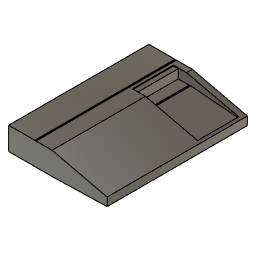
Basic shape (no keyboardd) hahahahahahah v1 (Autodesk Fusion 360 design; units mm, degrees)
Autodesk Fusion 360 part; units mm, degrees
sketch "Sketch1" plane through (0, 0, 0) normal (0, 1, 0) x (1, 0, 0)
  line L0 (0, 0) -> (0, -60.3)
  line L1 (0, 0) -> (115, 0)
  line L2 (0, -60.3) -> (115, -60.3)
  line L3 (261, -25.8907) -> (261, -3.8907)
  line L4 (115, 0) -> (261, -3.8907)
  line L5 (261, -25.8907) -> (115, -60.3)
  dimension "d1" = 60.3
  dimension "d2" = 115
  dimension "d3" = 115
  dimension "d4" = 150
  dimension "d5" = 22
  dimension "d6" = 146
  constraint coincident L0.start L1.start
  constraint vertical L0
  constraint perpendicular L0 L1
  constraint perpendicular L0 L2
  constraint vertical L3
  measures "d1" distance of L0.start L0.end
  measures "d2" distance of L0.start L1.end
  measures "d3" distance of L0.end L2.end
  measures "d4" distance of L2.end L3.start
  measures "d5" distance of L3.start L3.end
  measures "d6" horizontal distance of L1.end L3.end
extrude "Extrude1" add sketch "Sketch1" along normal blind 372
sketch "Sketch2" plane through (0, 0, 0) normal (0, -1, 0) x (1, 0, 0)
  line L0 (0, 60.3) -> (0, 0)
  line L1 (0, 0) -> (115, 0)
  line L2 (115, 0) -> (261, 3.8907)
  line L3 (261, 3.8907) -> (261, 25.8907)
  line L4 (261, 25.8907) -> (115, 60.3)
  line L5 (115, 60.3) -> (0, 60.3)
  line L6 (0, 0) -> (13.8, 0)
  line L7 (13.8, 0) -> (13.8, -2)
  line L8 (13.8, -2) -> (261.0312, -0.0411)
  line L9 (261, 3.8907) -> (261.0312, -0.0411)
  line L10 (261.0312, -0.0411) -> (247.2316, -0.1459)
  line L11 (247.2316, -0.1459) -> (247.1338, 3.5212)
  dimension "d9" = 13.8
  dimension "d10" = 2
  dimension "d11" = 13.8
  constraint coincident L0.end L1.start
  constraint perpendicular L0 L6
  constraint perpendicular L6 L7
  constraint coincident L2.end L3.start
  constraint coincident L8 L9.end
  constraint perpendicular L8 L9
  constraint coincident L2 L11.end
  constraint perpendicular L2 L11
  measures "d9" distance of L0.end L6.end
  measures "d10" distance of L6.end L7.end
  measures "d11" distance of L8.end L10.end
extrude "Extrude2" add sketch "Sketch2" against normal blind 358.2 contours L1 L2 L7 L8 L10 L11
extrude "Extrude3" cut sketch "Sketch2" against normal blind 13.8 contours L1 L2 L7 L8 L10 L11
sketch "Sketch3" plane through (0, 372, 0) normal (0, 1, 0) x (-1, 0, 0)
  line L0 (0, 0) -> (0, 60.3)
  line L1 (0, 60.3) -> (-115, 60.3)
  line L2 (-115, 60.3) -> (-261, 25.8907)
  line L3 (-261, 25.8907) -> (-261, 3.8907)
  line L4 (-261, 3.8907) -> (-115, 0)
  line L5 (-115, 0) -> (0, 0)
  line L6 (-115, 0) -> (0, 0)
  constraint coincident L4.end L5.start
  constraint coincident L0.start L5.end
extrude "Extrude5" cut 1 faces at (256.4313, 128.6, -0.076) along direction (0.007593, 0, -0.999971) blind 1.5
sketch "Sketch4" plane through (0.0167, 0, -2.1092) normal (0.007923, 0, -0.999969) x (0, 1, 0)
  line L0 (358.2, 247.2226) -> (13.8, 247.2226)
  line L1 (13.8, 247.2226) -> (13.8, 13.7837)
  line L2 (13.8, 13.7837) -> (358.2, 13.7837)
  line L3 (358.2, 13.7837) -> (358.2, 247.2226)
  line L4 (358.2, 13.7837) -> (350.3, 13.7837)
  line L5 (358.2, 13.7837) -> (358.2, 22.2837)
  line L6 (358.2, 22.2837) -> (350.3, 22.2837) construction
  line L7 (350.3, 13.7837) -> (350.3, 22.2837) construction
  line L8 (350.3, 22.2837) -> (326.3, 22.2837)
  line L9 (326.3, 22.2837) -> (326.3, 46.2837)
  line L10 (326.3, 46.2837) -> (350.3, 46.2837)
  line L11 (350.3, 46.2837) -> (350.3, 22.2837)
  line L12 (351.3, 21.2837) -> (325.3, 21.2837)
  line L13 (325.3, 21.2837) -> (325.3, 47.2837)
  line L14 (325.3, 47.2837) -> (351.3, 47.2837)
  line L15 (351.3, 47.2837) -> (351.3, 21.2837)
  line L16 (326.8, 45.7837) -> (349.8, 45.7837)
  line L17 (349.8, 45.7837) -> (349.8, 22.7837)
  line L18 (349.8, 22.7837) -> (326.8, 22.7837)
  line L19 (326.8, 22.7837) -> (326.8, 45.7837)
  line L20 (186, 13.7837) -> (186, 247.2226) construction
  line L21 (21.7, 22.2837) -> (45.7, 22.2837)
  line L22 (22.2, 22.7837) -> (45.2, 22.7837)
  line L23 (46.7, 47.2837) -> (20.7, 47.2837)
  line L24 (45.2, 22.7837) -> (45.2, 45.7837)
  line L25 (46.7, 21.2837) -> (46.7, 47.2837)
  line L26 (45.2, 45.7837) -> (22.2, 45.7837)
  line L27 (20.7, 47.2837) -> (20.7, 21.2837)
  line L28 (21.7, 46.2837) -> (21.7, 22.2837)
  line L29 (20.7, 21.2837) -> (46.7, 21.2837)
  line L30 (45.7, 46.2837) -> (21.7, 46.2837)
  line L31 (45.7, 22.2837) -> (45.7, 46.2837)
  line L32 (22.2, 45.7837) -> (22.2, 22.7837)
  line L33 (358.2, 130.5032) -> (13.8, 130.5032) construction
  line L34 (45.2, 238.2226) -> (45.2, 215.2226)
  line L35 (20.7, 213.7226) -> (20.7, 239.7226)
  line L36 (22.2, 238.2226) -> (45.2, 238.2226)
  line L37 (46.7, 213.7226) -> (20.7, 213.7226)
  line L38 (45.7, 238.7226) -> (45.7, 214.7226)
  line L39 (22.2, 215.2226) -> (22.2, 238.2226)
  line L40 (21.7, 238.7226) -> (45.7, 238.7226)
  line L41 (46.7, 239.7226) -> (46.7, 213.7226)
  line L42 (21.7, 214.7226) -> (21.7, 238.7226)
  line L43 (45.7, 214.7226) -> (21.7, 214.7226)
  line L44 (45.2, 215.2226) -> (22.2, 215.2226)
  line L45 (20.7, 239.7226) -> (46.7, 239.7226)
  line L46 (350.3, 214.7226) -> (350.3, 238.7226)
  line L47 (325.3, 239.7226) -> (325.3, 213.7226)
  line L48 (350.3, 238.7226) -> (326.3, 238.7226)
  line L49 (326.3, 214.7226) -> (350.3, 214.7226)
  line L50 (351.3, 213.7226) -> (351.3, 239.7226)
  line L51 (326.8, 215.2226) -> (349.8, 215.2226)
  line L52 (325.3, 213.7226) -> (351.3, 213.7226)
  line L53 (326.3, 238.7226) -> (326.3, 214.7226)
  line L54 (326.8, 238.2226) -> (326.8, 215.2226)
  line L55 (349.8, 238.2226) -> (326.8, 238.2226)
  line L56 (351.3, 239.7226) -> (325.3, 239.7226)
  line L57 (349.8, 215.2226) -> (349.8, 238.2226)
  dimension "d20" = 7.9
  dimension "d21" = 8.5
  dimension "d22" = 24
  dimension "d23" = 24
  dimension "d24" = -1
  dimension "d27" = 0.5
  constraint coincident L2.end L3.start
  constraint perpendicular L3 L4
  constraint perpendicular L4 L5
  constraint perpendicular L5 L6
  constraint coincident L6 L7.end
  constraint perpendicular L6 L7
  constraint horizontal L8
  constraint vertical L9
  constraint horizontal L10
  constraint vertical L11
  constraint midpoint L2 L20.start
  constraint midpoint L0 L20.end
  constraint symmetric L6.end L20 L21.start
  constraint symmetric L8.end L20 L21.end
  constraint symmetric L9.end L20 L30.start
  constraint symmetric L10.end L20 L28.start
  constraint symmetric L12.start L20 L27.end
  constraint symmetric L12.end L20 L25.start
  constraint symmetric L13.end L20 L23.start
  constraint symmetric L14.end L20 L23.end
  constraint symmetric L16.start L20 L24.end
  constraint symmetric L16.end L20 L26.end
  constraint symmetric L17.end L20 L22.start
  constraint symmetric L18.end L20 L22.end
  constraint midpoint L3 L33.start
  constraint midpoint L1 L33.end
  constraint symmetric L22.end L33 L34.start
  constraint symmetric L30.start L33 L38.end
  constraint symmetric L21.start L33 L40.start
  constraint symmetric L21.end L33 L38.start
  constraint symmetric L25.start L33 L41.start
  constraint symmetric L23.end L33 L35.start
  constraint symmetric L23.start L33 L37.start
  constraint symmetric L22.start L33 L36.start
  constraint symmetric L27.end L33 L35.end
  constraint symmetric L28.start L33 L42.start
  constraint symmetric L26.end L33 L39.start
  constraint symmetric L24.end L33 L34.end
  constraint symmetric L6.end L33 L46.end
  constraint symmetric L8.end L33 L48.end
  constraint symmetric L9.end L33 L49.start
  constraint symmetric L10.end L33 L46.start
  constraint symmetric L12.start L33 L50.end
  constraint symmetric L12.end L33 L47.start
  constraint symmetric L13.end L33 L47.end
  constraint symmetric L14.end L33 L50.start
  constraint symmetric L16.start L33 L51.start
  constraint symmetric L16.end L33 L51.end
  constraint symmetric L17.end L33 L55.start
  constraint symmetric L18.end L33 L54.start
  measures "d20" distance of L2.end L4.end
  measures "d21" distance of L2.end L5.end
  measures "d22" distance of L6.end L8.end
  measures "d23" distance of L6.end L10.end
extrude "Extrude8" add sketch "Sketch4" along normal blind 0.3 contours L12 L13 L14 L15 | L23 L25 L27 L29 | L35 L37 L41 L45 | L47 L50 L52 L56
extrude "Extrude9" add sketch "Sketch4" along normal blind 6 contours L16 L17 L18 L19 | L22 L24 L26 L32 | L34 L36 L39 L44 | L51 L54 L55 L57
fillet "Fillet2" radius 6 4 faces at (30.5137, 342.1333, -7.8678) (230.613, 334.4667, -6.2823) (222.9466, 29.8667, -6.3431) (30.5137, 37.5333, -7.8678)
sketch "Sketch5" plane through (19.5152, 0, 82.8039) normal (0.229395, 0, 0.973333) x (0, 1, 0)
  line L0 (0, -98.1008) -> (0, -248.1008)
  line L1 (0, -248.1008) -> (372, -248.1008)
  line L2 (372, -248.1008) -> (372, -98.1008)
  line L3 (372, -98.1008) -> (0, -98.1008)
  line L4 (372, -98.1008) -> (356.7, -98.1008)
  line L5 (356.7, -98.1008) -> (247.7, -98.1008)
  line L6 (247.7, -98.1008) -> (247.7, -248.1008)
  line L7 (356.7, -98.1008) -> (356.7, -248.1008)
  line L8 (247.7, -248.1008) -> (247.7, -240.1008)
  line L9 (247.7, -240.1008) -> (356.7, -240.1008)
  dimension "d38" = 15.3
  dimension "d39" = 109
  dimension "d40" = 8
  constraint coincident L2.end L3.start
  constraint perpendicular L2 L4
  constraint parallel L3 L5
  constraint coincident L1 L6.end
  constraint perpendicular L1 L6
  constraint coincident L1 L7.end
  constraint perpendicular L1 L7
  constraint perpendicular L1 L8
  constraint horizontal L9
  constraint coincident L7 L9.end
  measures "d38" distance of L2.end L4.end
  measures "d39" distance of L4.end L5.end
  measures "d40" distance of L6.end L8.end
sketch "Sketch6" plane through (0, 0, 60.3) normal (0, 0, 1) x (-1, 0, 0)
  line L0 (0, 0) -> (-115, 0)
  line L1 (-115, 0) -> (-115, -372)
  line L2 (-115, -372) -> (0, -372)
  line L3 (0, -372) -> (0, 0)
  line L4 (-115, -356.7) -> (-261, -356.7)
  line L5 (-115, -247.7) -> (-261, -247.7)
  line L6 (-253.2133, -247.7) -> (-253.2133, -356.7)
  line L7 (-115, -356.7) -> (-80.5, -356.7)
  line L8 (-115, -247.7) -> (-80.5, -247.7)
  line L9 (-80.5, -247.7) -> (-80.5, -356.7)
  dimension "d41" = 34.5
  dimension "d42" = 34.5
  constraint coincident L4.start L7.start
  constraint perpendicular L1 L7
  constraint coincident L5.start L8.start
  constraint perpendicular L1 L8
  measures "d41" distance of L4.start L7.end
  measures "d42" distance of L5.start L8.end
ref_plane "WorkPlane1" through (130.5, 356.7, 30.15) normal (0, 1, 0) x (0, 0, 1)
sketch "Sketch7" plane through (130.5, 356.7, 30.15) normal (0, 1, 0) x (1, 0, 0)
  line L0 (-15.5, -30.15) -> (130.5, 4.2593)
  line L1 (-15.5, -30.15) -> (130.5, 4.2593)
  line L2 (122.7133, 2.4241) -> (122.7133, 5.4241)
  line L3 (-15.5, -30.15) -> (-4.5013, -27.5578)
  line L4 (-130.5, -30.15) -> (-15.5, -30.15)
  line L5 (-4.5013, -27.5578) -> (-4.5013, -5.5578)
  line L6 (-4.5013, -5.5578) -> (122.7133, 5.4241)
  point P0 (122.7133, 2.4241)
  dimension "d44" = 3
  dimension "d45" = 11.3
  dimension "d46" = 22
  constraint coincident P0 L2.start
  constraint vertical L2
  constraint coincident L0.start L1.start
  constraint coincident L0 L3.end
  constraint perpendicular L4 L5
  measures "d44" distance of P0 L2.end
  measures "d45" distance of L0.start L3.end
  measures "d46" distance of L3.end L5.end
extrude "Extrude10" cut sketch "Sketch7" against normal blind 109
sketch "Sketch8" plane through (0, 0, 60.3) normal (0, 0, 1) x (-1, 0, 0)
  line L0 (0, 0) -> (-115, 0)
  line L1 (-115, 0) -> (-115, -372)
  line L2 (-115, -372) -> (0, -372)
  line L3 (0, -372) -> (0, 0)
  line L4 (-125.9987, -356.7) -> (-115, -356.7)
  line L5 (-125.9987, -247.7) -> (-115, -247.7)
  line L6 (-125.9987, -247.7) -> (-125.9987, -356.7)
  line L7 (-125.9987, -356.7) -> (-253.2133, -356.7)
  line L8 (-253.2133, -356.7) -> (-253.2133, -247.7)
  line L9 (-253.2133, -247.7) -> (-125.9987, -247.7)
  line L10 (-115, 0) -> (-261, 0)
  line L11 (-261, 0) -> (-261, -372)
  line L12 (-261, -372) -> (-115, -372)
  line L13 (-115, -372) -> (-115, 0)
  point P0 (-125.9987, -356.7)
  point P1 (-125.9987, -247.7)
  constraint coincident P0 L4.start
  constraint coincident L1 L4.end
  constraint perpendicular L1 L4
  constraint coincident P1 L5.start
  constraint coincident L1 L5.end
  constraint perpendicular L1 L5
extrude "Extrude11" cut sketch "Sketch8" against normal blind 25.5 contours L1 L4 L5 L6 L13
sketch "Sketch9" plane through (0, 0, 60.3) normal (0, 0, 1) x (-1, 0, 0)
  line L0 (0, 0) -> (-115, 0)
  line L1 (-115, 0) -> (-115, -247.7)
  line L2 (-115, -247.7) -> (-115, -356.7)
  line L3 (-115, -356.7) -> (-115, -372)
  line L4 (-115, -372) -> (0, -372)
  line L5 (0, -372) -> (0, 0)
  line L6 (-115, -356.7) -> (-93, -356.7)
  line L7 (-93, -356.7) -> (-80.5, -356.7)
  line L8 (-93, -356.7) -> (-93, -355.4342)
  line L9 (-93, -355.4342) -> (-93, -247.7)
  line L10 (-115, -247.7) -> (-80.5, -247.7)
  line L11 (-80.5, -356.7) -> (-80.5, -247.7)
  dimension "d51" = 22
  dimension "d52" = 12.5
  constraint coincident L2.end L3.start
  constraint perpendicular L3 L6
  constraint parallel L6 L7
  constraint perpendicular L7 L8
  constraint perpendicular L7 L9
  constraint coincident L1.end L2.start
  constraint perpendicular L9 L10
  constraint coincident L9.end L10
  constraint perpendicular L10 L11
  measures "d51" distance of L2.end L6.end
  measures "d52" distance of L6.end L7.end
extrude "Extrude12" cut sketch "Sketch9" against normal blind 25.5 contours L2 L6 L8 L9 L10
extrude "Extrude13" cut sketch "Sketch9" against normal blind 2 contours L7 L8 L9 L10 L11
sketch "Sketch10" plane through (0, 0, 34.8) normal (0, 0, 1) x (-1, 0, 0)
  line L0 (-125.9987, -247.7) -> (-125.9987, -356.7)
  line L1 (-125.9987, -356.7) -> (-93, -356.7)
  line L2 (-93, -356.7) -> (-93, -247.7)
  line L3 (-93, -247.7) -> (-125.9987, -247.7)
  line L4 (-125.9987, -356.7) -> (-121.9987, -356.7)
  line L5 (-121.9987, -356.7) -> (-121.9987, -247.7)
  dimension "d57" = 4
  constraint coincident L0.end L1.start
  constraint perpendicular L0 L4
  constraint vertical L5
  constraint coincident L3 L5.end
  measures "d57" distance of L0.end L4.end
extrude "Extrude14" add sketch "Sketch10" along normal blind 0.5 contours L0 L1 L3 L4 L5
sketch "Sketch11" plane through (0, 0, 60.3) normal (0, 0, 1) x (-1, 0, 0)
  line L0 (-115, -247.7) -> (-80.5, -247.7)
  line L1 (-80.5, -247.7) -> (-80.5, -356.7)
  line L2 (-80.5, -356.7) -> (-115, -356.7)
  line L3 (-115, -356.7) -> (-115, -372)
  line L4 (-115, -372) -> (0, -372)
  line L5 (0, -372) -> (0, 0)
  line L6 (0, 0) -> (-115, 0)
  line L7 (-115, 0) -> (-115, -247.7)
  line L8 (-115, 0) -> (-72, 0)
  line L9 (-72, 0) -> (-72, -372)
  line L10 (-72, 0) -> (-69, 0)
  line L11 (-69, 0) -> (-69, -372)
  dimension "d60" = 43
  dimension "d61" = 3
  constraint coincident L6.end L7.start
  constraint perpendicular L7 L8
  constraint coincident L4 L9.end
  constraint perpendicular L4 L9
  constraint perpendicular L9 L10
  constraint coincident L4 L11.end
  constraint perpendicular L4 L11
  measures "d60" distance of L6.end L8.end
  measures "d61" distance of L8.end L10.end
extrude "Extrude15" cut sketch "Sketch11" against normal blind 1 contours L4 L6 L9 L10 L11
